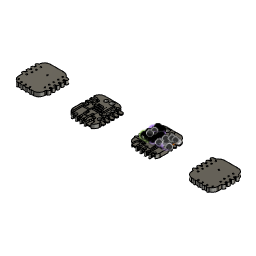
Coccinelle  Nano Paint Sensors v6 (Autodesk Fusion 360 design; units mm, degrees)
Autodesk Fusion 360 part; units mm, degrees
note: some values were not read from the file. Set by a fixed rule: which face or edge a step refers to.
(part 1 of 3)
sketch "Measure_ArduinoNano" plane through (0, 0, 0) normal (0, 0, 1) x (1, 0, 0)
  line L0 (-12.133, 30.8096) -> (-12.4229, 30.5196)
  arc A0 (-12.8135, 30.9102) -> (-12.8135, 31.1931) centre (-12.6721, 31.0517) cw
  line L1 (-12.5236, 31.2001) -> (-12.133, 30.8096)
  arc A1 (-4.5943, 42.68) -> (-4.5943, 42.08) centre (-4.2943, 42.38) ccw
  line L2 (-11.771, 0) -> (-6.771, 0)
  line L3 (-13.9477, 42.68) -> (-13.7477, 42.88)
  line L4 (0, 0) -> (0, 43.18)
  line L5 (-12.4229, 30.5196) -> (-12.8135, 30.9102)
  line L6 (-1.524, 21.656) -> (-1.024, 21.656)
  arc A2 (-4.7943, 41.88) -> (-6.271, 41.88) centre (-5.5326, 41.1416) ccw
  line L7 (-13.9477, 37.28) -> (-13.7477, 37.48)
  line L8 (-6.0616, 30.4622) -> (-6.3515, 30.7521)
  line L9 (-4.5417, 27.9093) -> (-9.0003, 23.4507)
  line L10 (-12.0199, 1.0002) -> (-10.4999, 1.0002)
  line L11 (-6.8307, 32.0124) -> (-7.2212, 31.6218)
  line L12 (-11.6107, 25.028) -> (-12.0012, 24.6374)
  line L13 (-1.524, 36.656) -> (-1.024, 36.656)
  arc A3 (-6.8307, 32.2953) -> (-6.8307, 32.0124) centre (-6.9721, 32.1539) cw
  arc A4 (-7.1206, 32.3023) -> (-6.8377, 32.3023) centre (-6.9791, 32.1609) cw
  circle A5 centre (-7.271, 3.0017) radius 0.76
  circle A6 centre (-1.524, 4.156) radius 0.5
  circle A7 centre (-17.018, 14.156) radius 0.5
  circle A8 centre (-17.018, 19.156) radius 0.5
  line L14 (-5.671, 30.8528) -> (-6.0616, 30.4622)
  line L15 (-6.3515, 30.7521) -> (-5.9609, 31.1427)
  line L16 (-12.2912, 24.9274) -> (-11.9006, 25.3179)
  line L17 (-11.771, 18.0694) -> (-6.771, 18.0694)
  line L18 (-11.9006, 25.3179) -> (-11.6107, 25.028)
  line L19 (-12.4635, 0) -> (-12.4635, 4.2)
  circle A9 centre (-1.524, 6.656) radius 0.889
  arc A10 (-12.0012, 24.6374) -> (-12.2841, 24.6374) centre (-12.1427, 24.7789) cw
  line L20 (-17.018, 12.156) -> (-17.018, 11.156)
  line L21 (-8.0618, 33.5265) -> (-7.9903, 33.4549)
  circle A11 centre (-1.524, 36.656) radius 0.889
  line L22 (-12.2841, 24.6374) -> (-12.2912, 24.6445)
  line L23 (0, 43.18) -> (-6.271, 43.18)
  circle A12 centre (-1.524, 24.156) radius 0.889
  line L24 (-6.771, 13.9686) -> (-11.771, 13.9686)
  line L25 (-8.7353, 33.1359) -> (-8.3447, 33.5265)
  circle A13 centre (-17.018, 11.656) radius 0.889
  circle A14 centre (-17.018, 4.156) radius 0.5
  line L26 (-6.771, 18.0694) -> (-6.771, 13.9686)
  circle A15 centre (-1.524, 6.656) radius 0.5
  circle A16 centre (-17.018, 16.656) radius 0.5
  line L27 (-1.524, 19.156) -> (-1.024, 19.156)
  circle A17 centre (-17.018, 9.156) radius 0.5
  line L28 (-7.271, 0.2361) -> (-7.271, 1.7561)
  circle A18 centre (-17.018, 19.156) radius 0.889
  line L29 (-6.8377, 32.3023) -> (-6.8307, 32.2953)
  line L30 (-7.2212, 31.6218) -> (-7.5112, 31.9118)
  arc A19 (-9.0003, 23.4507) -> (-9.1417, 23.3921) centre (-9.1417, 23.5921) cw
  line L31 (-8.3809, 32.7815) -> (-8.7353, 33.1359)
  circle A20 centre (-1.524, 19.156) radius 0.5
  arc A21 (-5.9609, 31.1427) -> (-5.6781, 31.1427) centre (-5.8195, 31.0013) cw
  line L32 (-9.0003, 32.9093) -> (-4.5417, 28.4507)
  circle A22 centre (-7.271, 0.9961) radius 0.76
  arc A23 (-4.5417, 28.4507) -> (-4.4831, 28.3093) centre (-4.6831, 28.3093) cw
  circle A24 centre (-1.524, 9.156) radius 0.889
  arc A25 (-7.9903, 33.4549) -> (-7.9903, 33.1721) centre (-8.1317, 33.3135) cw
  line L33 (-17.518, 11.656) -> (-16.518, 11.656)
  line L34 (-7.9903, 33.1721) -> (-8.3809, 32.7815)
  line L35 (-4.4831, 28.3093) -> (-4.4831, 28.0507)
  arc A26 (-9.4003, 23.3921) -> (-9.5417, 23.4507) centre (-9.4003, 23.5921) cw
  circle A27 centre (-17.018, 6.656) radius 0.889
  circle A28 centre (-17.018, 6.656) radius 0.5
  circle A29 centre (-9.271, 3) radius 0.76
  circle A30 centre (-17.018, 14.156) radius 0.889
  arc A31 (-9.5417, 32.9093) -> (-9.4003, 32.9678) centre (-9.4003, 32.7678) cw
  arc A32 (-4.4831, 28.0507) -> (-4.5417, 27.9093) centre (-4.6831, 28.0507) cw
  line L36 (-9.1417, 23.3921) -> (-9.4003, 23.3921)
  arc A33 (-5.671, 31.1356) -> (-5.671, 30.8528) centre (-5.8124, 30.9942) cw
  line L37 (-11.771, 13.9686) -> (-11.771, 18.0694)
  arc A34 (-8.3447, 33.5265) -> (-8.0618, 33.5265) centre (-8.2033, 33.385) cw
  line L38 (-7.5112, 31.9118) -> (-7.1206, 32.3023)
  line L39 (-9.4003, 32.9678) -> (-9.1417, 32.9678)
  line L40 (-18.542, 43.18) -> (-18.542, 0)
  line L41 (-12.4635, 4.2) -> (-6.0786, 4.2)
  circle A35 centre (-1.524, 16.656) radius 0.5
  circle A36 centre (-1.524, 24.156) radius 0.5
  line L42 (-12.271, 42.88) -> (-12.271, 43.18)
  line L43 (-12.271, 41.88) -> (-13.7477, 41.88)
  line L44 (-13.7477, 41.88) -> (-13.9477, 42.08)
  line L45 (-1.524, 24.156) -> (-1.024, 24.156)
  line L46 (-6.0786, 4.2) -> (-6.0786, 0)
  arc A37 (-13.7477, 37.48) -> (-12.271, 37.48) centre (-13.0093, 38.2183) ccw
  line L47 (-6.271, 36.48) -> (-6.271, 36.18)
  line L48 (-12.271, 36.18) -> (-12.271, 36.48)
  arc A38 (-13.7477, 42.88) -> (-12.271, 42.88) centre (-13.0093, 43.6183) ccw
  line L49 (-6.271, 42.88) -> (-4.7943, 42.88)
  arc A39 (-4.5943, 37.28) -> (-4.5943, 36.68) centre (-4.2943, 36.98) ccw
  circle A40 centre (-17.018, 16.656) radius 0.889
  line L50 (-4.5943, 36.68) -> (-4.7943, 36.48)
  arc A41 (-4.7943, 36.48) -> (-6.271, 36.48) centre (-5.5326, 35.7416) ccw
  line L51 (-4.7943, 42.88) -> (-4.5943, 42.68)
  line L52 (-6.271, 37.48) -> (-4.7943, 37.48)
  line L53 (-18.542, 43.18) -> (0, 43.18)
  line L54 (-13.7477, 36.48) -> (-13.9477, 36.68)
  line L55 (-6.771, 0) -> (0, 0)
  line L56 (-12.271, 36.48) -> (-13.7477, 36.48)
  line L57 (-6.271, 43.18) -> (-6.271, 42.88)
  line L58 (-7.771, 0.9965) -> (-6.511, 0.9965)
  circle A42 centre (-17.018, 11.656) radius 0.5
  line L59 (-6.271, 36.18) -> (-12.271, 36.18)
  line L60 (-12.271, 43.18) -> (-18.542, 43.18)
  line L61 (-4.5943, 42.08) -> (-4.7943, 41.88)
  circle A43 centre (-1.524, 14.156) radius 0.5
  line L62 (-16.518, 19.156) -> (-17.018, 19.156)
  line L63 (-4.7943, 37.48) -> (-4.5943, 37.28)
  circle A44 centre (-17.018, 31.656) radius 0.889
  line L64 (-12.271, 37.48) -> (-12.271, 41.88)
  line L65 (-6.271, 41.88) -> (-6.271, 37.48)
  line L66 (-15.829, 4.2) -> (-2.8014, 4.2)
  line L67 (-12.8135, 31.1931) -> (-12.8065, 31.2001)
  line L68 (-18.542, 0) -> (-11.771, 0)
  line L69 (-6.0786, 0) -> (-12.4635, 0)
  circle A45 centre (-1.524, 9.156) radius 0.5
  arc A46 (-13.9477, 36.68) -> (-13.9477, 37.28) centre (-14.2477, 36.98) ccw
  line L70 (0, 43.18) -> (-18.542, 43.18)
  circle A47 centre (-1.524, 16.656) radius 0.889
  arc A48 (-13.9477, 42.08) -> (-13.9477, 42.68) centre (-14.2477, 42.38) ccw
  circle A49 centre (-1.524, 14.156) radius 0.889
  arc A50 (-12.8065, 31.2001) -> (-12.5236, 31.2001) centre (-12.665, 31.0587) cw
  circle A51 centre (-1.524, 11.656) radius 0.5
  circle A52 centre (-17.018, 9.156) radius 0.889
  arc A53 (-9.1417, 32.9678) -> (-9.0003, 32.9093) centre (-9.1417, 32.7678) cw
  arc A54 (-12.2912, 24.6445) -> (-12.2912, 24.9274) centre (-12.1497, 24.7859) cw
  arc A55 (-5.7285, 25.4497) -> (-5.7285, 25.1669) centre (-5.8699, 25.3083) cw
  line L71 (-5.6781, 31.1427) -> (-5.671, 31.1356)
  arc A56 (-5.7355, 25.1598) -> (-6.0184, 25.1598) centre (-5.8769, 25.3012) cw
  arc A57 (-6.5407, 31.7225) -> (-6.2579, 31.7225) centre (-6.3993, 31.5811) cw
  line L72 (-6.0184, 25.1598) -> (-6.409, 25.5504)
  circle A58 centre (-11.269, 3) radius 0.76
  line L73 (-8.4384, 23.521) -> (-8.0478, 23.1304)
  line L74 (-8.3447, 22.8335) -> (-8.7353, 23.2241)
  line L75 (-6.5982, 24.58) -> (-6.9888, 24.9706)
  line L76 (-7.178, 24.0002) -> (-7.5686, 24.3907)
  line L77 (-7.2787, 24.6807) -> (-6.8881, 24.2901)
  line L78 (-6.6414, 31.042) -> (-6.9313, 31.3319)
  arc A59 (-13.1609, 25.7971) -> (-13.4437, 25.7971) centre (-13.3023, 25.9385) cw
  line L79 (-7.8011, 32.2017) -> (-8.091, 32.4916)
  line L80 (-5.4385, 25.7396) -> (-5.8291, 26.1302)
  circle A60 centre (-1.524, 36.656) radius 0.5
  line L81 (-5.8291, 26.1302) -> (-5.5392, 26.4201)
  circle A61 centre (-1.524, 4.156) radius 0.889
  circle A62 centre (-17.018, 34.156) radius 0.889
  line L82 (-7.4105, 32.5923) -> (-7.8011, 32.2017)
  line L83 (-14.0589, 28.0507) -> (-14.0589, 28.3093)
  arc A63 (-8.0618, 22.8335) -> (-8.3447, 22.8335) centre (-8.2033, 22.9749) cw
  line L84 (-17.518, 6.656) -> (-16.518, 6.656)
  arc A64 (-7.7004, 32.8822) -> (-7.4176, 32.8822) centre (-7.559, 32.7408) cw
  line L85 (-1.524, 34.156) -> (-1.024, 34.156)
  line L86 (-1.524, 39.156) -> (-1.024, 39.156)
  line L87 (-6.2579, 31.7225) -> (-6.2508, 31.7154)
  arc A65 (-6.3083, 24.8699) -> (-6.3083, 24.5871) centre (-6.4497, 24.7285) cw
  line L88 (-6.6989, 25.2605) -> (-6.3083, 24.8699)
  arc A66 (-5.1486, 26.0296) -> (-5.1486, 25.7467) centre (-5.2901, 25.8881) cw
  line L89 (-8.091, 32.4916) -> (-7.7004, 32.8822)
  circle A67 centre (-1.524, 39.156) radius 0.889
  line L90 (-6.3083, 24.5871) -> (-6.3154, 24.58)
  line L91 (-5.5392, 26.4201) -> (-5.1486, 26.0296)
  circle A68 centre (-1.524, 34.156) radius 0.5
  line L92 (-8.7353, 23.2241) -> (-8.4384, 23.521)
  line L93 (-6.8881, 24.0072) -> (-6.8952, 24.0002)
  line L94 (-6.409, 25.5504) -> (-6.119, 25.8403)
  line L95 (-14.0003, 28.4507) -> (-9.5417, 32.9093)
  arc A69 (-14.0589, 28.3093) -> (-14.0003, 28.4507) centre (-13.8589, 28.3093) cw
  line L96 (-7.4176, 32.8822) -> (-7.4105, 32.8751)
  arc A70 (-7.4105, 32.8751) -> (-7.4105, 32.5923) centre (-7.5519, 32.7337) cw
  line L97 (-13.4508, 26.087) -> (-13.0602, 26.4776)
  line L98 (-6.2508, 31.4326) -> (-6.6414, 31.042)
  line L99 (-13.6401, 27.0574) -> (-13.3501, 26.7675)
  arc A71 (-14.6175, 26.9708) -> (-14.6175, 27.2537) centre (-14.4761, 27.1122) cw
  arc A72 (-13.7407, 26.3769) -> (-14.0236, 26.3769) centre (-13.8822, 26.5183) cw
  arc A73 (-6.3154, 24.58) -> (-6.5982, 24.58) centre (-6.4568, 24.7214) cw
  line L100 (-6.9888, 24.9706) -> (-6.6989, 25.2605)
  arc A74 (-5.0912, 30.5558) -> (-5.0912, 30.2729) centre (-5.2326, 30.4144) cw
  line L101 (-7.7579, 23.4203) -> (-8.1484, 23.8109)
  arc A75 (-5.1557, 25.7396) -> (-5.4385, 25.7396) centre (-5.2971, 25.8811) cw
  line L102 (-3.9245, 26.9708) -> (-3.996, 26.8993)
  line L103 (-14.0306, 26.6668) -> (-13.6401, 27.0574)
  line L104 (-13.4437, 25.7971) -> (-13.4508, 25.8042)
  line L105 (-5.2493, 26.7101) -> (-4.9594, 27)
  line L106 (-12.7703, 26.1877) -> (-13.1609, 25.7971)
  line L107 (-1.524, 29.156) -> (-1.024, 29.156)
  line L108 (-5.7285, 25.1669) -> (-5.7355, 25.1598)
  line L109 (-5.4818, 29.8824) -> (-5.7717, 30.1723)
  line L110 (-7.8585, 24.1008) -> (-7.4679, 23.7102)
  line L111 (-4.9019, 29.3025) -> (-5.1918, 29.5924)
  line L112 (-14.6034, 26.9568) -> (-14.6175, 26.9708)
  arc A76 (-14.0306, 26.384) -> (-14.0306, 26.6668) centre (-13.8892, 26.5254) cw
  line L113 (-13.0602, 26.4776) -> (-12.7703, 26.1877)
  circle A77 centre (-1.524, 26.656) radius 0.889
  line L114 (-11.8431, 31.0995) -> (-12.2337, 31.4901)
  line L115 (-17.018, 37.156) -> (-17.018, 36.156)
  line L116 (-6.119, 25.8403) -> (-5.7285, 25.4497)
  arc A78 (-8.0478, 23.1304) -> (-8.0478, 22.8476) centre (-8.1892, 22.989) cw
  arc A79 (-4.5688, 26.6094) -> (-4.5688, 26.3265) centre (-4.7102, 26.468) cw
  circle A80 centre (-11.2599, 1.0002) radius 0.76
  circle A81 centre (-1.524, 31.656) radius 0.5
  line L117 (-8.0478, 22.8476) -> (-8.0618, 22.8335)
  line L118 (-3.9386, 29.4032) -> (-3.9245, 29.3891)
  line L119 (-11.364, 32.3598) -> (-10.9734, 31.9692)
  line L120 (-4.3151, 27.6443) -> (-3.9245, 27.2537)
  arc A82 (-7.475, 23.4203) -> (-7.7579, 23.4203) centre (-7.6164, 23.5618) cw
  line L121 (-4.6695, 27.2899) -> (-4.3151, 27.6443)
  circle A83 centre (-1.524, 29.156) radius 0.889
  arc A84 (-11.6539, 32.0699) -> (-11.6539, 32.3527) centre (-11.5125, 32.2113) cw
  arc A85 (-14.0003, 27.9093) -> (-14.0589, 28.0507) centre (-13.8589, 28.0507) cw
  line L122 (-1.524, 26.656) -> (-1.024, 26.656)
  line L123 (-4.8587, 26.3195) -> (-5.2493, 26.7101)
  line L124 (-4.2789, 26.8993) -> (-4.6695, 27.2899)
  line L125 (-14.0236, 26.3769) -> (-14.0306, 26.384)
  arc A86 (-4.2214, 29.4032) -> (-3.9386, 29.4032) centre (-4.08, 29.2618) cw
  arc A87 (-5.3811, 30.5629) -> (-5.0982, 30.5629) centre (-5.2397, 30.4214) cw
  line L126 (-9.5417, 23.4507) -> (-14.0003, 27.9093)
  arc A88 (-3.996, 26.8993) -> (-4.2789, 26.8993) centre (-4.1375, 27.0407) cw
  arc A89 (-13.4508, 25.8042) -> (-13.4508, 26.087) centre (-13.3094, 25.9456) cw
  line L127 (-7.5686, 24.3907) -> (-7.2787, 24.6807)
  line L128 (-6.9313, 31.3319) -> (-6.5407, 31.7225)
  line L129 (-13.3501, 26.7675) -> (-13.7407, 26.3769)
  circle A90 centre (-1.524, 29.156) radius 0.5
  line L130 (-11.5532, 31.3894) -> (-11.8431, 31.0995)
  circle A91 centre (-1.524, 26.656) radius 0.5
  arc A92 (-6.8952, 24.0002) -> (-7.178, 24.0002) centre (-7.0366, 24.1416) cw
  arc A93 (-6.8881, 24.2901) -> (-6.8881, 24.0072) centre (-7.0295, 24.1486) cw
  arc A94 (-6.2508, 31.7154) -> (-6.2508, 31.4326) centre (-6.3922, 31.574) cw
  line L131 (-10.9734, 31.9692) -> (-11.2633, 31.6793)
  circle A95 centre (-17.018, 26.656) radius 0.5
  line L132 (-8.1484, 23.8109) -> (-7.8585, 24.1008)
  line L133 (-9.8067, 33.1359) -> (-10.1036, 32.839)
  line L134 (-7.4679, 23.4274) -> (-7.475, 23.4203)
  arc A96 (-10.4801, 33.5265) -> (-10.1973, 33.5265) centre (-10.3387, 33.385) cw
  line L135 (-5.0982, 30.5629) -> (-5.0912, 30.5558)
  arc A97 (-4.5759, 26.3195) -> (-4.8587, 26.3195) centre (-4.7173, 26.4609) cw
  line L136 (-13.9732, 30.0334) -> (-13.9661, 30.0405)
  circle A98 centre (-17.018, 36.656) radius 0.5
  line L137 (-17.518, 36.656) -> (-16.518, 36.656)
  arc A99 (-11.6468, 32.3598) -> (-11.364, 32.3598) centre (-11.5054, 32.2184) cw
  line L138 (-14.6175, 27.2537) -> (-14.2269, 27.6443)
  circle A100 centre (-1.524, 34.156) radius 0.9737
  line L139 (-5.7717, 30.1723) -> (-5.3811, 30.5629)
  line L140 (-4.3151, 28.7157) -> (-4.612, 29.0126)
  arc A101 (-11.1315, 23.4849) -> (-11.1315, 23.7677) centre (-10.9901, 23.6263) cw
  line L141 (-16.518, 26.656) -> (-17.018, 26.656)
  line L142 (-11.9438, 31.78) -> (-11.5532, 31.3894)
  arc A102 (-4.8013, 29.983) -> (-4.5184, 29.983) centre (-4.6598, 29.8416) cw
  line L143 (-11.2633, 31.6793) -> (-11.6539, 32.0699)
  line L144 (-4.5688, 26.3265) -> (-4.5759, 26.3195)
  line L145 (-11.6539, 32.3527) -> (-11.6468, 32.3598)
  line L146 (-5.0912, 30.2729) -> (-5.4818, 29.8824)
  line L147 (-4.9594, 27) -> (-4.5688, 26.6094)
  arc A103 (-3.9245, 29.3891) -> (-3.9245, 29.1063) centre (-4.0659, 29.2477) cw
  line L148 (-5.1486, 25.7467) -> (-5.1557, 25.7396)
  arc A104 (-14.3206, 26.9568) -> (-14.6034, 26.9568) centre (-14.462, 27.0982) cw
  arc A105 (-7.4679, 23.7102) -> (-7.4679, 23.4274) centre (-7.6094, 23.5688) cw
  line L149 (-5.1918, 29.5924) -> (-4.8013, 29.983)
  line L150 (-1.524, 31.656) -> (-1.024, 31.656)
  line L151 (-16.518, 21.656) -> (-17.018, 21.656)
  line L152 (-10.3935, 32.549) -> (-10.6835, 32.2591)
  arc A106 (-4.5113, 29.976) -> (-4.5113, 29.6931) centre (-4.6528, 29.8345) cw
  arc A107 (-3.9245, 27.2537) -> (-3.9245, 26.9708) centre (-4.0659, 27.1122) cw
  line L153 (-13.93, 27.3473) -> (-14.3206, 26.9568)
  line L154 (-4.5184, 29.983) -> (-4.5113, 29.976)
  line L155 (-14.2269, 27.6443) -> (-13.93, 27.3473)
  line L156 (-4.5113, 29.6931) -> (-4.9019, 29.3025)
  circle A108 centre (-17.018, 29.156) radius 0.5
  circle A109 centre (-17.018, 31.656) radius 0.5
  arc A110 (-11.067, 32.9396) -> (-10.7841, 32.9396) centre (-10.9256, 32.7982) cw
  line L157 (-10.1036, 32.839) -> (-10.4942, 33.2295)
  circle A111 centre (-17.018, 24.156) radius 0.5
  arc A112 (-14.5459, 29.4607) -> (-14.2631, 29.4607) centre (-14.4045, 29.3192) cw
  arc A113 (-13.9661, 30.0405) -> (-13.6833, 30.0405) centre (-13.8247, 29.8991) cw
  arc A114 (-12.5811, 25.2173) -> (-12.8639, 25.2173) centre (-12.7225, 25.3587) cw
  line L158 (-4.612, 29.0126) -> (-4.2214, 29.4032)
  line L159 (-16.518, 29.156) -> (-17.018, 29.156)
  circle A115 centre (-17.018, 36.656) radius 0.889
  circle A116 centre (-17.018, 34.156) radius 0.5
  circle A117 centre (-17.018, 39.156) radius 0.889
  circle A118 centre (-1.524, 39.156) radius 0.5
  line L160 (-10.6835, 32.2591) -> (-11.0741, 32.6497)
  line L161 (-13.2927, 29.6499) -> (-13.5826, 29.36)
  line L162 (-10.4942, 33.5124) -> (-10.4801, 33.5265)
  line L163 (-12.4804, 25.8978) -> (-12.1905, 25.6079)
  line L164 (-13.3934, 30.6132) -> (-13.3863, 30.6203)
  circle A119 centre (-17.018, 39.156) radius 0.5
  circle A120 centre (-17.018, 29.156) radius 0.889
  arc A121 (-12.871, 25.2243) -> (-12.871, 25.5072) centre (-12.7296, 25.3658) cw
  line L165 (-3.9245, 29.1063) -> (-4.3151, 28.7157)
  arc A122 (-10.8416, 23.4778) -> (-11.1244, 23.4778) centre (-10.983, 23.6192) cw
  arc A123 (-14.6175, 29.1063) -> (-14.6175, 29.3891) centre (-14.4761, 29.2477) cw
  line L166 (-13.0028, 29.9398) -> (-13.3934, 30.3304)
  line L167 (-11.0741, 32.9326) -> (-11.067, 32.9396)
  line L168 (-14.2269, 28.7157) -> (-14.6175, 29.1063)
  line L169 (-10.1973, 33.5265) -> (-9.8067, 33.1359)
  arc A124 (-13.3863, 30.6203) -> (-13.1034, 30.6203) centre (-13.2449, 30.4789) cw
  circle A125 centre (-1.524, 21.656) radius 0.889
  line L170 (-10.4801, 22.8335) -> (-10.5517, 22.905)
  arc A126 (-11.0741, 32.6497) -> (-11.0741, 32.9326) centre (-10.9326, 32.7911) cw
  line L171 (-14.6175, 29.3891) -> (-14.5459, 29.4607)
  line L172 (-12.1905, 25.6079) -> (-12.5811, 25.2173)
  line L173 (-10.7409, 24.1583) -> (-10.451, 23.8684)
  line L174 (-13.5826, 29.36) -> (-13.9732, 29.7506)
  line L175 (-10.7841, 32.9396) -> (-10.3935, 32.549)
  arc A127 (-13.3934, 30.3304) -> (-13.3934, 30.6132) centre (-13.2519, 30.4718) cw
  circle A128 centre (-17.018, 24.156) radius 0.889
  circle A129 centre (-17.018, 26.656) radius 0.889
  line L176 (-12.8639, 25.2173) -> (-12.871, 25.2243)
  line L177 (-13.8725, 29.0701) -> (-14.2269, 28.7157)
  line L178 (-11.1315, 23.7677) -> (-10.7409, 24.1583)
  arc A130 (-10.4942, 33.2295) -> (-10.4942, 33.5124) centre (-10.3528, 33.371) cw
  line L179 (-12.871, 25.5072) -> (-12.4804, 25.8978)
  arc A131 (-13.9732, 29.7506) -> (-13.9732, 30.0334) centre (-13.8318, 29.892) cw
  line L180 (-11.1244, 23.4778) -> (-11.1315, 23.4849)
  line L181 (-16.518, 24.156) -> (-17.018, 24.156)
  line L182 (-12.2337, 31.7729) -> (-12.2266, 31.78)
  line L183 (-13.6833, 30.0405) -> (-13.2927, 29.6499)
  line L184 (-14.2631, 29.4607) -> (-13.8725, 29.0701)
  line L185 (-13.1034, 30.6203) -> (-12.7129, 30.2297)
  arc A132 (-12.2266, 31.78) -> (-11.9438, 31.78) centre (-12.0852, 31.6386) cw
  line L186 (-12.7129, 30.2297) -> (-13.0028, 29.9398)
  arc A133 (-12.2337, 31.4901) -> (-12.2337, 31.7729) centre (-12.0923, 31.6315) cw
  arc A134 (-11.4214, 24.0576) -> (-11.7043, 24.0576) centre (-11.5628, 24.199) cw
  line L187 (-11.7113, 24.3475) -> (-11.3207, 24.7381)
  circle A135 centre (-17.018, 21.656) radius 0.889
  circle A136 centre (-1.524, 21.656) radius 0.5
  line L188 (-11.0308, 24.4482) -> (-11.4214, 24.0576)
  circle A137 centre (-17.018, 21.656) radius 0.5
  line L189 (-15.829, 4.2) -> (-15.829, 43.18)
  line L190 (-10.451, 23.8684) -> (-10.8416, 23.4778)
  line L191 (-11.7043, 24.0576) -> (-11.7113, 24.0647)
  line L192 (-10.5517, 23.1879) -> (-10.1611, 23.5785)
  line L193 (-10.1611, 23.5785) -> (-9.8067, 23.2241)
  line L194 (0, 43.18) -> (0, 0)
  circle A138 centre (-1.524, 31.656) radius 0.9737
  arc A139 (-10.1973, 22.8335) -> (-10.4801, 22.8335) centre (-10.3387, 22.9749) cw
  circle A140 centre (-9.271, 0.998) radius 0.76
  line L195 (-16.518, 14.156) -> (-17.018, 14.156)
  line L196 (-9.8067, 23.2241) -> (-10.1973, 22.8335)
  line L197 (-11.3207, 24.7381) -> (-11.0308, 24.4482)
  line L198 (-18.542, 0) -> (-18.542, 43.18)
  arc A141 (-11.7113, 24.0647) -> (-11.7113, 24.3475) centre (-11.5699, 24.2061) cw
  circle A142 centre (-1.524, 19.156) radius 0.889
  line L199 (-2.024, 11.656) -> (-1.024, 11.656)
  line L200 (-2.8014, 4.2) -> (-2.8014, 43.18)
  circle A143 centre (-1.524, 11.656) radius 0.889
  line L201 (-16.518, 16.656) -> (-17.018, 16.656)
  circle A144 centre (-17.018, 4.156) radius 0.889
  arc A145 (-10.5517, 22.905) -> (-10.5517, 23.1879) centre (-10.4103, 23.0465) cw
sketch "Sketch2" plane through (0, 0, 0) normal (0, 0, 1) x (1, 0, 0)
  line L0 (-1.524, 39.156) -> (-1.024, 39.156) construction
  line L1 (-17.018, 39.156) -> (-1.524, 39.156) construction
  line L2 (-1.524, 36.656) -> (-11.7254, 36.6745) construction
  line L3 (-11.7254, 36.6745) -> (-11.73, 34.156) construction
  line L4 (-11.73, 34.156) -> (-1.524, 34.156) construction
  line L5 (-15.829, 4.2) -> (-15.829, 43.18)
  line L6 (-1.524, 31.656) -> (-17.018, 31.656) construction
  line L7 (-1.524, 29.156) -> (-1.024, 29.156) construction
  line L8 (-17.018, 29.156) -> (-1.524, 29.156) construction
  line L9 (-1.524, 26.656) -> (-17.018, 26.656) construction
  line L10 (-1.524, 24.156) -> (-1.024, 24.156) construction
  line L11 (-17.018, 24.156) -> (-1.524, 24.156) construction
  line L12 (-1.524, 21.656) -> (-17.018, 21.656) construction
  line L13 (-17.018, 19.156) -> (-1.524, 19.156) construction
  line L14 (-2.8014, 4.2) -> (-2.8014, 43.18)
  line L15 (-1.524, 14.156) -> (-11.0509, 14.156) construction
  line L16 (-11.0509, 14.156) -> (-11.0509, 16.656) construction
  line L17 (-11.0509, 16.656) -> (-1.524, 16.656) construction
  point P0 (-17.018, 39.156)
  point P1 (-1.524, 39.156)
  point P2 (-1.524, 36.656)
  point P3 (-1.524, 34.156)
  point P4 (-1.524, 31.656)
  point P5 (-17.018, 31.656)
  point P6 (-17.018, 29.156)
  point P7 (-1.524, 29.156)
  point P8 (-1.524, 26.656)
  point P9 (-17.018, 26.656)
  point P10 (-17.018, 24.156)
  point P11 (-1.524, 24.156)
  point P12 (-1.524, 21.656)
  point P13 (-17.018, 21.656)
  point P14 (-17.018, 19.156)
  point P15 (-1.524, 19.156)
  point P16 (-1.524, 16.656)
  point P17 (-17.018, 16.656)
  point P18 (-1.524, 14.156)
  constraint coincident P0 L1.start
  constraint coincident P1 L0.start
  constraint coincident P2 L2.start
  constraint perpendicular L2 L3
  constraint coincident P3 L4.end
  constraint horizontal L4
  constraint coincident P4 L6.start
  constraint coincident P5 L6.end
  constraint coincident P6 L8.start
  constraint coincident P7 L7.start
  constraint coincident P8 L9.start
  constraint coincident P9 L9.end
  constraint coincident P10 L11.start
  constraint coincident P11 L10.start
  constraint coincident P12 L12.start
  constraint coincident P13 L12.end
  constraint coincident P14 L13.start
  constraint coincident P15 L13.end
  constraint coincident P18 L15.start
  constraint perpendicular L14 L15
  constraint perpendicular L15 L16
  constraint coincident P16 L17.end
  constraint perpendicular L16 L17
sketch "Sketch3" plane through (0, 0, 0) normal (0, 0, 1) x (1, 0, 0)
  line L0 (-101.7185, 80.6951) -> (98.6412, 80.6951)
  line L1 (98.6412, 80.6951) -> (98.6412, -44.7509)
  line L2 (98.6412, -44.7509) -> (-101.7185, -44.7509)
  line L3 (-101.7185, -44.7509) -> (-101.7185, 80.6951)
  constraint horizontal L0
  constraint vertical L1
  constraint horizontal L2
  constraint vertical L3
extrude "Extrude1" add sketch "Sketch3" against normal blind 8.7 makes body 1
sketch "Top" plane through (0, 0, 0) normal (0, 0, 1) x (1, 0, 0)
  line L0 (-17.0187, 17.631) -> (-2.5746, 17.6243)
  arc A0 (-2.5746, 17.6243) -> (-2.5732, 20.6743) centre (-2.5739, 19.1493) ccw
  line L1 (-2.5732, 20.6743) -> (-17.0173, 20.681)
  arc A1 (-17.0173, 20.681) -> (-17.0187, 17.631) centre (-17.018, 19.156) ccw
  line L2 (-17.018, 19.156) -> (-2.5739, 19.1493) construction
  line L3 (-17.0185, 22.631) -> (-1.6713, 22.6262)
  arc A2 (-1.6713, 22.6262) -> (-1.6704, 25.6762) centre (-1.6709, 24.1512) ccw
  line L4 (-1.6704, 25.6762) -> (-17.0175, 25.681)
  arc A3 (-17.0175, 25.681) -> (-17.0185, 22.631) centre (-17.018, 24.156) ccw
  line L5 (-17.018, 24.156) -> (-1.6709, 24.1512) construction
  line L6 (-17.0184, 27.631) -> (-1.671, 27.6268)
  arc A4 (-1.671, 27.6268) -> (-1.6701, 30.6768) centre (-1.6705, 29.1518) ccw
  line L7 (-1.6701, 30.6768) -> (-17.0176, 30.681)
  arc A5 (-17.0176, 30.681) -> (-17.0184, 27.631) centre (-17.018, 29.156) ccw
  line L8 (-17.018, 29.156) -> (-1.6705, 29.1518) construction
  line L9 (-17.0183, 37.631) -> (-1.6707, 37.6278)
  arc A6 (-1.6707, 37.6278) -> (-1.6701, 40.6778) centre (-1.6704, 39.1528) ccw
  line L10 (-1.6701, 40.6778) -> (-17.0177, 40.681)
  arc A7 (-17.0177, 40.681) -> (-17.0183, 37.631) centre (-17.018, 39.156) ccw
  line L11 (-17.018, 39.156) -> (-1.6704, 39.1528) construction
  line L12 (-11.7302, 32.631) -> (-1.6714, 32.6293)
  arc A8 (-1.6714, 32.6293) -> (-1.6709, 35.6793) centre (-1.6711, 34.1543) ccw
  line L13 (-1.6709, 35.6793) -> (-11.7297, 35.681)
  arc A9 (-11.7297, 35.681) -> (-11.7302, 32.631) centre (-11.73, 34.156) ccw
  line L14 (-11.73, 34.156) -> (-1.6711, 34.1543) construction
  line L15 (-32.018, 39.1539) -> (-17.018, 39.156) construction
  line L16 (11.8289, 34.1518) -> (-1.6711, 34.1543) construction
  line L17 (-17.018, 29.156) -> (-32.018, 29.1601) construction
  line L18 (-1.6709, 24.1512) -> (11.8289, 24.1466) construction
  line L19 (-24.8881, 39.1549) -> (-24.8908, 29.1581) construction
  line L20 (-24.8908, 29.1581) -> (-28.224, 19.1614) construction
  line L21 (-28.224, 19.1614) -> (-28.2258, 9.1646) construction
  line L22 (-17.018, 19.156) -> (-6.0959, 19.1509) construction
  line L23 (-32.018, 9.1646) -> (-24.596, 9.1646) construction
  line L24 (-24.596, 9.1646) -> (-24.596, 19.1564) construction
  line L25 (-24.596, 19.1564) -> (-17.018, 19.156) construction
  point P0 (-17.018, 19.156)
  point P1 (-17.018, 24.156)
  point P2 (-17.018, 29.156)
  point P3 (-17.018, 39.156)
  point P4 (-11.73, 34.156)
  point P5 (-11.0509, 14.156)
  dimension "d9" = 3.05
  dimension "d10" = 3.05
  dimension "d11" = 3.05
  dimension "d12" = 3.05
  dimension "d18" = 3.05
  dimension "d37" = 15
  dimension "d38" = 9.9968
  dimension "d39" = 9.9968
  dimension "d40" = 9.9968
  constraint tangent L0 A0
  constraint tangent A0 L1
  constraint parallel L0 L1
  constraint tangent L1 A1
  constraint tangent L0 A1
  constraint coincident P0 A1.centre
  constraint tangent L3 A2
  constraint tangent A2 L4
  constraint parallel L3 L4
  constraint tangent L4 A3
  constraint tangent L3 A3
  constraint coincident P1 A3.centre
  constraint tangent L6 A4
  constraint tangent A4 L7
  constraint parallel L6 L7
  constraint tangent L7 A5
  constraint tangent L6 A5
  constraint coincident P2 A5.centre
  constraint tangent L9 A6
  constraint tangent A6 L10
  constraint parallel L9 L10
  constraint tangent L10 A7
  constraint tangent L9 A7
  constraint coincident P3 A7.centre
  constraint tangent L12 A8
  constraint tangent A8 L13
  constraint parallel L12 L13
  constraint tangent L13 A9
  constraint tangent L12 A9
  constraint coincident P4 A9.centre
  constraint coincident A8.centre L14.end
  constraint parallel L8 L17
  constraint coincident A2.centre L5.end
  constraint coincident L15 L19.start
  constraint coincident L17 L19.end
  constraint perpendicular L17 L19
  constraint parallel L2 L22
  constraint horizontal L23
  constraint perpendicular L23 L24
  measures "d9" diameter of A0
  measures "d10" diameter of A2
  measures "d11" diameter of A4
  measures "d12" diameter of A6
  measures "d18" diameter of A8
  measures "d37" horizontal distance of L15.start P3
  measures "d38" vertical distance of L19.start L19.end
  measures "d39" vertical distance of L19.end L20.end
  measures "d40" vertical distance of L20.end L21.end
sketch "Down" plane through (0, 0, 0) normal (0, 0, 1) x (1, 0, 0)
  line L0 (-17.0184, 30.131) -> (4.8275, 30.125)
  arc A0 (4.8275, 30.125) -> (4.8283, 33.175) centre (4.8279, 31.65) ccw
  line L1 (4.8283, 33.175) -> (-17.0176, 33.181)
  arc A1 (-17.0176, 33.181) -> (-17.0184, 30.131) centre (-17.018, 31.656) ccw
  line L2 (-17.018, 31.656) -> (4.8279, 31.65) construction
  line L3 (-1.6701, 30.6768) -> (-17.0176, 30.681)
  line L4 (-17.0186, 25.131) -> (-2.1697, 25.1252)
  arc A2 (-2.1697, 25.1252) -> (-2.1685, 28.1752) centre (-2.1691, 26.6502) ccw
  line L5 (-2.1685, 28.1752) -> (-17.0174, 28.181)
  arc A3 (-17.0174, 28.181) -> (-17.0186, 25.131) centre (-17.018, 26.656) ccw
  line L6 (-17.018, 26.656) -> (4.8309, 26.65) construction
  line L7 (-17.019, 20.131) -> (-2.1714, 20.1215)
  arc A4 (-2.1714, 20.1215) -> (-2.1695, 23.1715) centre (-2.1705, 21.6465) ccw
  line L8 (-2.1695, 23.1715) -> (-17.017, 23.181)
  arc A5 (-17.017, 23.181) -> (-17.019, 20.131) centre (-17.018, 21.656) ccw
  line L9 (-17.018, 21.656) -> (-2.1705, 21.6465) construction
  line L10 (-11.7258, 35.1495) -> (-2.1716, 35.1473)
  arc A6 (-2.1716, 35.1473) -> (-2.1708, 38.1973) centre (-2.1712, 36.6723) ccw
  line L11 (-2.1708, 38.1973) -> (-11.7251, 38.1995)
  arc A7 (-11.7251, 38.1995) -> (-11.7258, 35.1495) centre (-11.7254, 36.6745) ccw
  line L12 (-11.7254, 36.6745) -> (-2.1712, 36.6723) construction
  line L13 (4.8279, 31.65) -> (6.3519, 31.6496)
  line L14 (4.8279, 31.65) -> (6.3519, 31.6496)
  line L15 (-1.6709, 24.1512) -> (11.8289, 24.1466)
  line L16 (18.1446, 34.1486) -> (18.1412, 24.1445) construction
  line L17 (18.1446, 34.1486) -> (18.148, 44.1528) construction
  line L18 (-23.6867, 26.6539) -> (-17.018, 26.656) construction
  line L19 (-17.018, 29.156) -> (-32.018, 29.1601)
  line L20 (-32.018, 39.1539) -> (-17.018, 39.156)
  line L21 (-29.9727, 29.1595) -> (-29.974, 39.1542) construction
  line L22 (-29.974, 39.1542) -> (-29.975, 49.1489) construction
  line L23 (-23.6867, 26.6539) -> (-23.6898, 49.151) construction
  arc A8 (-32.0179, 29.6233) -> (-32.018, 29.1601) centre (-32.0179, 29.3917) ccw construction
  line L24 (-23.6898, 49.151) -> (-32.018, 49.1502) construction
  line L25 (-29.9727, 29.1595) -> (-29.9754, 19.1648) construction
  line L26 (-32.018, 19.1617) -> (-23.6867, 19.1628) construction
  line L27 (-23.6867, 19.1628) -> (-23.6862, 21.656) construction
  line L28 (-23.6862, 21.656) -> (-17.018, 21.656) construction
  point P0 (-17.018, 31.656)
  point P1 (-17.018, 26.656)
  point P2 (-17.018, 21.656)
  point P3 (-11.0509, 16.656)
  point P4 (-11.7254, 36.6745)
  dimension "d13" = 3.05
  dimension "d14" = 3.05
  dimension "d15" = 3.05
  dimension "d17" = 3.05
  constraint tangent L0 A0
  constraint tangent A0 L1
  constraint parallel L0 L1
  constraint tangent L1 A1
  constraint tangent L0 A1
  constraint parallel L2 L3
  constraint coincident P0 A1.centre
  constraint tangent L4 A2
  constraint tangent A2 L5
  constraint parallel L4 L5
  constraint tangent L5 A3
  constraint tangent L4 A3
  constraint parallel L0 L6
  constraint coincident P1 A3.centre
  constraint tangent L7 A4
  constraint tangent A4 L8
  constraint parallel L7 L8
  constraint tangent L8 A5
  constraint tangent L7 A5
  constraint coincident P2 A5.centre
  constraint tangent L10 A6
  constraint tangent A6 L11
  constraint parallel L10 L11
  constraint tangent L11 A7
  constraint tangent L10 A7
  constraint coincident P4 A7.centre
  constraint coincident A0.centre L2.end
  constraint parallel L13 L14
  constraint coincident L15 L16.end
  constraint perpendicular L15 L16
  constraint equal L16 L17
  constraint coincident L19 L21.start
  constraint coincident L20 L21.end
  constraint perpendicular L20 L21
  constraint equal L21 L22
  constraint perpendicular L20 L23
  constraint coincident L19.end A8.end
  constraint tangent L19 A8
  constraint perpendicular L22 L24
  constraint perpendicular L19 L25
  constraint equal L21 L25
  constraint perpendicular L23 L26
  constraint horizontal L28
  measures "d13" diameter of A0
  measures "d14" diameter of A2
  measures "d15" diameter of A4
  measures "d17" diameter of A6
sketch "Middle" plane through (0, 0, 0) normal (0, 0, 1) x (1, 0, 0)
  line L0 (-11.0509, 14.156) -> (-11.0509, 16.656)
  circle A0 centre (-11.7277, 35.4153) radius 1.525
  line L1 (-11.7254, 36.6745) -> (-11.73, 34.156)
  dimension "d21" = 3.05
  constraint midpoint A0.centre L1
  measures "d21" diameter of A0
sketch "PinHoles" plane through (0, 0, 0) normal (0, 0, 1) x (1, 0, 0)
  circle A0 centre (-1.524, 39.156) radius 0.45
  circle A1 centre (-1.524, 36.656) radius 0.45
  circle A2 centre (-1.524, 34.156) radius 0.45
  circle A3 centre (-1.524, 31.656) radius 0.45
  circle A4 centre (-1.524, 29.156) radius 0.45
  circle A5 centre (-1.524, 26.656) radius 0.45
  circle A6 centre (-1.524, 24.156) radius 0.45
  circle A7 centre (-1.524, 21.656) radius 0.45
  circle A8 centre (-1.524, 19.156) radius 0.45
  circle A9 centre (-1.524, 16.656) radius 0.45
  circle A10 centre (-1.524, 14.156) radius 0.45
  circle A11 centre (-1.524, 11.656) radius 0.45
  circle A12 centre (-1.524, 9.156) radius 0.45
  circle A13 centre (-1.524, 6.656) radius 0.45
  circle A14 centre (-1.524, 4.156) radius 0.45
  circle A15 centre (-7.271, 3.0017) radius 0.45
  circle A16 centre (-7.271, 0.9961) radius 0.45
  circle A17 centre (-9.271, 0.998) radius 0.45
  circle A18 centre (-9.271, 3) radius 0.45
  circle A19 centre (-11.2599, 1.0002) radius 0.45
  circle A20 centre (-11.269, 3) radius 0.45
  circle A21 centre (-17.018, 4.156) radius 0.45
  circle A22 centre (-17.018, 6.656) radius 0.45
  circle A23 centre (-17.018, 9.156) radius 0.45
  circle A24 centre (-17.018, 11.656) radius 0.45
  circle A25 centre (-17.018, 14.156) radius 0.45
  circle A26 centre (-17.018, 16.656) radius 0.45
  circle A27 centre (-17.018, 19.156) radius 0.45
  circle A28 centre (-17.018, 21.656) radius 0.45
  circle A29 centre (-17.018, 24.156) radius 0.45
  circle A30 centre (-17.018, 26.656) radius 0.45
  circle A31 centre (-17.018, 29.156) radius 0.45
  circle A32 centre (-17.018, 31.656) radius 0.45
  circle A33 centre (-17.018, 34.156) radius 0.45
  circle A34 centre (-17.018, 36.656) radius 0.45
  circle A35 centre (-17.018, 39.156) radius 0.45
  point P0 (-1.524, 39.156)
  point P1 (-1.524, 36.656)
  point P2 (-1.524, 34.156)
  point P3 (-1.524, 31.656)
  point P4 (-1.524, 29.156)
  point P5 (-1.524, 26.656)
  point P6 (-1.524, 24.156)
  point P7 (-1.524, 21.656)
  point P8 (-1.524, 19.156)
  point P9 (-1.524, 16.656)
  point P10 (-1.524, 14.156)
  point P11 (-1.524, 11.656)
  point P12 (-1.524, 9.156)
  point P13 (-1.524, 6.656)
  point P14 (-1.524, 4.156)
  point P15 (-7.271, 3.0017)
  point P16 (-7.271, 0.9961)
  point P17 (-9.271, 0.998)
  point P18 (-9.271, 3)
  point P19 (-11.2599, 1.0002)
  point P20 (-11.269, 3)
  point P21 (-17.018, 4.156)
  point P22 (-17.018, 6.656)
  point P23 (-17.018, 9.156)
  point P24 (-17.018, 11.656)
  point P25 (-17.018, 14.156)
  point P26 (-17.018, 16.656)
  point P27 (-17.018, 19.156)
  point P28 (-17.018, 21.656)
  point P29 (-17.018, 24.156)
  point P30 (-17.018, 26.656)
  point P31 (-17.018, 29.156)
  point P32 (-17.018, 31.656)
  point P33 (-17.018, 34.156)
  point P34 (-17.018, 36.656)
  point P35 (-17.018, 39.156)
  dimension "d22" = 0.9
  constraint coincident P0 A0.centre
  constraint coincident P1 A1.centre
  constraint coincident P2 A2.centre
  constraint coincident P3 A3.centre
  constraint coincident P4 A4.centre
  constraint coincident P5 A5.centre
  constraint coincident P6 A6.centre
  constraint coincident P7 A7.centre
  constraint coincident P8 A8.centre
  constraint coincident P9 A9.centre
  constraint coincident P10 A10.centre
  constraint coincident P11 A11.centre
  constraint coincident P12 A12.centre
  constraint coincident P13 A13.centre
  constraint coincident P14 A14.centre
  constraint coincident P15 A15.centre
  constraint coincident P16 A16.centre
  constraint coincident P17 A17.centre
  constraint coincident P18 A18.centre
  constraint coincident P19 A19.centre
  constraint coincident P20 A20.centre
  constraint coincident P21 A21.centre
  constraint coincident P22 A22.centre
  constraint coincident P23 A23.centre
  constraint coincident P24 A24.centre
  constraint coincident P25 A25.centre
  constraint coincident P26 A26.centre
  constraint coincident P27 A27.centre
  constraint coincident P28 A28.centre
  constraint coincident P29 A29.centre
  constraint coincident P30 A30.centre
  constraint coincident P31 A31.centre
  constraint coincident P32 A32.centre
  constraint coincident P33 A33.centre
  constraint coincident P34 A34.centre
  constraint equal A0 A1
  constraint coincident P35 A35.centre
  constraint equal A0 A35
  constraint equal A34 A35
  constraint equal A33 A35
  constraint equal A32 A35
  constraint equal A31 A35
  constraint equal A30 A35
  constraint equal A29 A35
  constraint equal A28 A35
  constraint equal A27 A35
  constraint equal A26 A35
  constraint equal A25 A35
  constraint equal A24 A35
  constraint equal A23 A35
  constraint equal A22 A35
  constraint equal A21 A35
  constraint equal A0 A2
  constraint equal A0 A3
  constraint equal A0 A4
  constraint equal A0 A5
  constraint equal A0 A6
  constraint equal A0 A7
  constraint equal A0 A8
  constraint equal A0 A9
  constraint equal A0 A10
  constraint equal A0 A11
  constraint equal A0 A15
  constraint equal A0 A12
  constraint equal A0 A13
  constraint equal A0 A14
  constraint equal A15 A18
  constraint equal A15 A20
  constraint equal A15 A19
  constraint equal A15 A17
  constraint equal A15 A16
  measures "d22" diameter of A0
extrude "Extrude2" add sketch "Top" against normal blind 2.7 separate body makes body 2 at (-6.7864, 24.6611, 0) makes body 3 at (-11.902, 39.6632, 0) makes body 4 at (-7.3888, 18.6432, 0) makes body 5 at (-6.7865, 28.6448, 0) makes body 6 at (-5.0242, 33.6465, 0)
combine "Combine1" operation cut target body 1 tool bodies 2 4 5 3 6
extrude "Extrude3" add sketch "Down" along normal blind 4 separate body makes body 7 at (-12.0689, 25.1291, 1.3333) makes body 8 at (-2.4536, 33.177, 2.6667) makes body 9 at (-7.1187, 23.1747, 1.3333) makes body 10 at (-5.3556, 38.198, 1.3333)
move_body "Move2" bodies 10 7 8 9 to x (1, 0, 0) y (0, 1, 0) z (0, 0, 1) at (0, 0, -8.7)
combine "Combine2" operation cut target body 1 tool bodies 7 10 8 9
extrude "Extrude4" cut sketch "Middle" against normal blind 8.7 bodies 1
extrude "Extrude5" cut sketch "PinHoles" against normal blind 8.7 bodies 1
sketch "TopTunnels" plane through (0, 0, 0) normal (0, 0, 1) x (1, 0, 0)
  line L0 (-17.0182, 40.681) -> (-32.0182, 40.679)
  arc A0 (-32.0182, 40.679) -> (-32.0178, 37.6289) centre (-32.018, 39.1539) ccw
  line L1 (-32.0178, 37.6289) -> (-17.0178, 37.6309)
  arc A1 (-17.0178, 37.6309) -> (-17.0182, 40.681) centre (-17.018, 39.156) ccw
  line L2 (-17.018, 39.156) -> (-32.018, 39.1539) construction
  line L3 (-32.018, 39.1539) -> (-17.018, 39.156)
  line L4 (-17.0176, 30.6809) -> (-32.0176, 30.685)
  arc A2 (-32.0176, 30.685) -> (-32.0184, 27.6352) centre (-32.018, 29.1601) ccw
  line L5 (-32.0184, 27.6352) -> (-17.0184, 27.6311)
  arc A3 (-17.0184, 27.6311) -> (-17.0176, 30.6809) centre (-17.018, 29.156) ccw
  line L6 (-17.018, 29.156) -> (-32.018, 29.1601) construction
  line L7 (-1.6714, 32.6293) -> (11.8286, 32.6268)
  arc A4 (11.8286, 32.6268) -> (11.8292, 35.6768) centre (11.8289, 34.1518) ccw
  line L8 (11.8292, 35.6768) -> (-1.6708, 35.6793)
  arc A5 (-1.6708, 35.6793) -> (-1.6714, 32.6293) centre (-1.6711, 34.1543) ccw
  line L9 (-1.6711, 34.1543) -> (11.8289, 34.1518) construction
  line L10 (-1.6714, 22.6262) -> (11.8284, 22.6216)
  arc A6 (11.8284, 22.6216) -> (11.8294, 25.6716) centre (11.8289, 24.1466) ccw
  line L11 (11.8294, 25.6716) -> (-1.6703, 25.6762)
  arc A7 (-1.6703, 25.6762) -> (-1.6714, 22.6262) centre (-1.6709, 24.1512) ccw
  line L12 (-1.6709, 24.1512) -> (11.8289, 24.1466) construction
  line L13 (-17.0179, 20.7691) -> (-24.5959, 20.7696)
  arc A8 (-24.5959, 20.7696) -> (-24.596, 17.5433) centre (-24.596, 19.1564) ccw
  line L14 (-24.596, 17.5433) -> (-17.0181, 17.5428)
  arc A9 (-17.0181, 17.5428) -> (-17.0179, 20.7691) centre (-17.018, 19.156) ccw
  line L15 (-17.018, 19.156) -> (-24.596, 19.1564) construction
  line L16 (-26.121, 19.1564) -> (-26.121, 9.1646)
  arc A10 (-26.121, 9.1646) -> (-23.071, 9.1646) centre (-24.596, 9.1646) ccw
  line L17 (-23.071, 9.1646) -> (-23.071, 19.1564)
  arc A11 (-23.071, 19.1564) -> (-26.121, 19.1564) centre (-24.596, 19.1564) ccw
  line L18 (-24.596, 19.1564) -> (-24.596, 9.1646) construction
  line L19 (-24.596, 10.7778) -> (-32.018, 10.7778)
  arc A12 (-32.018, 10.7778) -> (-32.018, 7.5514) centre (-32.018, 9.1646) ccw
  line L20 (-32.018, 7.5514) -> (-24.596, 7.5514)
  arc A13 (-24.596, 7.5514) -> (-24.596, 10.7778) centre (-24.596, 9.1646) ccw
  line L21 (-24.596, 9.1646) -> (-32.018, 9.1646) construction
  point P0 (-17.018, 39.156)
  point P1 (-32.018, 39.1539)
  point P2 (-17.018, 29.156)
  point P3 (-32.018, 29.1601)
  point P4 (-1.6711, 34.1543)
  point P5 (11.8289, 34.1518)
  point P6 (-1.6709, 24.1512)
  point P7 (11.8289, 24.1466)
  point P8 (-1.6727, 14.1517)
  point P9 (11.8289, 14.1509)
  point P10 (-17.018, 19.156)
  point P11 (-24.596, 19.1564)
  point P12 (-24.596, 9.1646)
  point P13 (-32.018, 9.1646)
  constraint tangent L0 A0
  constraint tangent A0 L1
  constraint parallel L0 L1
  constraint tangent L1 A1
  constraint tangent L0 A1
  constraint coincident P1 A0.centre
  constraint parallel L2 L3
  constraint coincident P0 A1.centre
  constraint tangent L4 A2
  constraint tangent A2 L5
  constraint parallel L4 L5
  constraint tangent L5 A3
  constraint tangent L4 A3
  constraint coincident P3 A2.centre
  constraint coincident P2 A3.centre
  constraint tangent L7 A4
  constraint tangent A4 L8
  constraint parallel L7 L8
  constraint tangent L8 A5
  constraint tangent L7 A5
  constraint coincident P5 A4.centre
  constraint coincident P4 A5.centre
  constraint tangent L10 A6
  constraint tangent A6 L11
  constraint parallel L10 L11
  constraint tangent L11 A7
  constraint tangent L10 A7
  constraint coincident P7 A6.centre
  constraint coincident P6 A7.centre
  constraint tangent L13 A8
  constraint tangent A8 L14
  constraint parallel L13 L14
  constraint tangent L14 A9
  constraint tangent L13 A9
  constraint coincident P11 A8.centre
  constraint coincident P10 A9.centre
  constraint tangent L16 A10
  constraint tangent A10 L17
  constraint parallel L16 L17
  constraint tangent L17 A11
  constraint tangent L16 A11
  constraint coincident P12 A10.centre
  constraint vertical L18
  constraint tangent L19 A12
  constraint tangent A12 L20
  constraint parallel L19 L20
  constraint tangent L20 A13
  constraint tangent L19 A13
  constraint coincident P13 A12.centre
  constraint perpendicular L16 L21
sketch "DownTunnels" plane through (0, 0, 0) normal (0, 0, 1) x (1, 0, 0)
  line L0 (-17.018, 23.181) -> (-23.6862, 23.181)
  arc A0 (-23.6862, 23.181) -> (-23.6862, 20.131) centre (-23.6862, 21.656) ccw
  line L1 (-23.6862, 20.131) -> (-17.018, 20.131)
  arc A1 (-17.018, 20.131) -> (-17.018, 23.181) centre (-17.018, 21.656) ccw
  line L2 (-17.018, 21.656) -> (-23.6862, 21.656) construction
  line L3 (-23.6862, 21.656) -> (-17.018, 21.656)
  line L4 (-25.2112, 21.6563) -> (-25.2117, 19.1633)
  arc A2 (-25.2117, 19.1633) -> (-22.1617, 19.1627) centre (-23.6867, 19.163) ccw
  line L5 (-22.1617, 19.1627) -> (-22.1612, 21.6557)
  arc A3 (-22.1612, 21.6557) -> (-25.2112, 21.6563) centre (-23.6862, 21.656) ccw
  line L6 (-23.6862, 21.656) -> (-23.6867, 19.163) construction
  line L7 (-23.6868, 20.688) -> (-32.0181, 20.6872)
  arc A4 (-32.0181, 20.6872) -> (-32.0178, 17.6372) centre (-32.018, 19.1622) ccw
  line L8 (-32.0178, 17.6372) -> (-23.6865, 17.638)
  arc A5 (-23.6865, 17.638) -> (-23.6868, 20.688) centre (-23.6867, 19.163) ccw
  line L9 (-23.6867, 19.163) -> (-32.018, 19.1622) construction
  line L10 (-32.018, 19.1617) -> (-23.6867, 19.1628)
  line L11 (-17.0185, 28.181) -> (-23.6871, 28.1789)
  arc A6 (-23.6871, 28.1789) -> (-23.6862, 25.1289) centre (-23.6867, 26.6539) ccw
  line L12 (-23.6862, 25.1289) -> (-17.0175, 25.131)
  arc A7 (-17.0175, 25.131) -> (-17.0185, 28.181) centre (-17.018, 26.656) ccw
  line L13 (-17.018, 26.656) -> (-23.6867, 26.6539) construction
  line L14 (-23.6867, 26.6539) -> (-17.018, 26.656)
  line L15 (-22.1617, 26.654) -> (-22.1638, 49.1512)
  arc A8 (-22.1638, 49.1512) -> (-25.2138, 49.1509) centre (-23.6888, 49.151) ccw
  line L16 (-25.2138, 49.1509) -> (-25.2117, 26.6537)
  arc A9 (-25.2117, 26.6537) -> (-22.1617, 26.654) centre (-23.6867, 26.6539) ccw
  line L17 (-23.6867, 26.6539) -> (-23.6888, 49.151) construction
  line L18 (-23.689, 50.676) -> (-32.0181, 50.6752)
  arc A10 (-32.0181, 50.6752) -> (-32.0178, 47.6252) centre (-32.018, 49.1502) ccw
  line L19 (-32.0178, 47.6252) -> (-23.6887, 47.626)
  arc A11 (-23.6887, 47.626) -> (-23.689, 50.676) centre (-23.6888, 49.151) ccw
  line L20 (-23.6888, 49.151) -> (-32.018, 49.1502) construction
  line L21 (6.3529, 31.6496) -> (6.3563, 44.1572)
  arc A12 (6.3563, 44.1572) -> (3.3063, 44.158) centre (4.8313, 44.1576) ccw
  line L22 (3.3063, 44.158) -> (3.3029, 31.6504)
  arc A13 (3.3029, 31.6504) -> (6.3529, 31.6496) centre (4.8279, 31.65) ccw
  line L23 (4.84, 42.6326) -> (12.1811, 42.6744)
  arc A14 (12.1811, 42.6744) -> (12.1638, 45.7243) centre (12.1724, 44.1993) ccw
  line L24 (12.1638, 45.7243) -> (4.8227, 45.6826)
  arc A15 (4.8227, 45.6826) -> (4.84, 42.6326) centre (4.8313, 44.1576) ccw
  line L25 (4.8279, 31.65) -> (4.8313, 44.1576) construction
  line L26 (-17.018, 31.656) -> (4.8279, 31.65)
  line L27 (4.8313, 44.1576) -> (12.1724, 44.1993)
  point P0 (-17.018, 21.656)
  point P1 (-23.6862, 21.656)
  point P2 (-23.6867, 19.1628)
  point P3 (-32.018, 19.1617)
  point P4 (-17.018, 26.656)
  point P5 (-23.6867, 26.6539)
  point P6 (-23.6898, 49.151)
  point P7 (-32.018, 49.1502)
  point P8 (4.8279, 31.65)
  constraint tangent L0 A0
  constraint tangent A0 L1
  constraint parallel L0 L1
  constraint tangent L1 A1
  constraint tangent L0 A1
  constraint coincident P1 A0.centre
  constraint parallel L2 L3
  constraint coincident P0 A1.centre
  constraint tangent L4 A2
  constraint tangent A2 L5
  constraint parallel L4 L5
  constraint tangent L5 A3
  constraint tangent L4 A3
  constraint coincident A2.centre P2
  constraint tangent L7 A4
  constraint tangent A4 L8
  constraint parallel L7 L8
  constraint tangent L8 A5
  constraint tangent L7 A5
  constraint coincident A4.centre P3
  constraint parallel L9 L10
  constraint coincident A2.centre L6.end
  constraint tangent L11 A6
  constraint tangent A6 L12
  constraint parallel L11 L12
  constraint tangent L12 A7
  constraint tangent L11 A7
  constraint coincident P5 A6.centre
  constraint parallel L13 L14
  constraint coincident P4 A7.centre
  constraint tangent L15 A8
  constraint tangent A8 L16
  constraint parallel L15 L16
  constraint tangent L16 A9
  constraint tangent L15 A9
  constraint coincident A8.centre P6
  constraint tangent L18 A10
  constraint tangent A10 L19
  constraint parallel L18 L19
  constraint tangent L19 A11
  constraint tangent L18 A11
  constraint coincident P7 A10.centre
  constraint perpendicular L17 L20
  constraint coincident P6 A8.centre
  constraint tangent L21 A12
  constraint tangent A12 L22
  constraint parallel L21 L22
  constraint tangent L22 A13
  constraint tangent L21 A13
  constraint tangent L23 A14
  constraint tangent A14 L24
  constraint parallel L23 L24
  constraint tangent L24 A15
  constraint tangent L23 A15
  constraint coincident P8 A13.centre
  constraint coincident A12.centre A15.centre
  constraint perpendicular L25 L26
  constraint coincident A14.centre L27.end
extrude "Extrude6" add sketch "TopTunnels" against normal blind 2.7 separate body makes body 11 at (-21.5616, 19.694, 0) makes body 12 at (2.829, 34.6618, 0) makes body 13 at (-27.0181, 39.663, 0) makes body 14 at (-27.0179, 29.667, 0) makes body 15 at (2.8289, 23.6413, 0)
combine "Combine3" operation cut target body 1 tool bodies 11 15 14 12 13
extrude "Extrude7" add sketch "DownTunnels" along normal blind 4 separate body makes body 16 at (-26.9719, 18.6544, 0) makes body 17 at (-24.1957, 34.153, 0) makes body 18 at (4.3217, 39.4832, 0)
move_body "Move3" bodies 18 16 17 to x (1, 0, 0) y (0, 1, 0) z (0, 0, 1) at (0, 0, -8.7)
combine "Combine4" operation cut target body 1 tool bodies 16 18 17